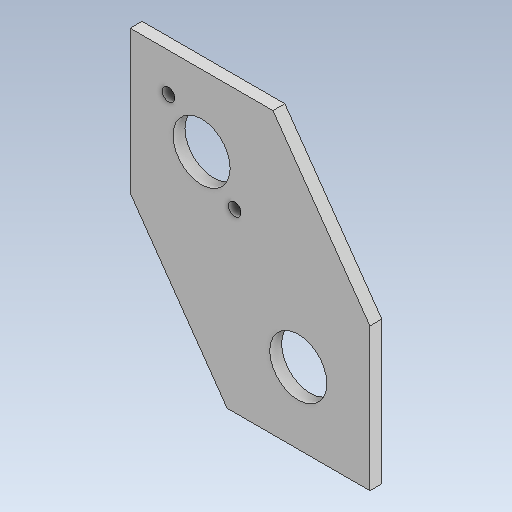
# Autodesk Inventor part: Motor and gearbox panel
Saved by Autodesk Inventor 2020.2 (Build 242310000, 310)
## iProperties
Created: 2020-02-27
Part Number: Motor and gearbox panel
Material: Generic
Document SubType Name: Modeling
Designer: deli
Density: 1 g/cm^3
Appearance: Default
Author: deli
Autodesk Inventor part; units mm, degrees
ref_plane "YZ Plane" through (0, 0, 0) normal (1, 0, 0) x (0, 1, 0)
ref_plane "XZ Plane" through (0, 0, 0) normal (0, 1, 0) x (-1, 0, 0)
ref_plane "XY Plane" through (0, 0, 0) normal (0, 0, 1) x (1, 0, 0)
sketch "Sketch1" plane through (0, 0, 0) normal (0, 0, 1) x (1, 0, 0)
  circle A0 centre (30.5438, 1.69) radius 1.7
  circle A1 centre (48.2215, -15.9877) radius 1.7
  line L0 (20.3327, -25.9449) -> (20.3327, 11.6471) projected
  circle A2 centre (39.3827, -7.1489) radius 7.62
  line L1 (39.3827, -7.1489) -> (121.2052, -7.1489) construction
  line L2 (20.3327, 11.9011) -> (58.4327, 11.9011)
  line L3 (39.3827, -7.1489) -> (118.6167, -7.1489) construction
  circle A3 centre (65.1936, -44.0106) radius 7.62
  line L4 (20.3327, 11.9011) -> (90.1827, 11.9011)
  line L5 (90.1827, 11.9011) -> (90.1827, -64.2989)
  line L6 (90.1827, -64.2989) -> (20.3327, -64.2989)
  line L7 (20.3327, -64.2989) -> (20.3327, 11.9011)
  circle A4 centre (65.1936, -44.0106) radius 18.9992
  line L8 (39.3827, -7.1489) -> (98.3795, -91.4051)
  line L9 (39.3827, -7.1489) -> (142.2405, -7.1489) construction
  line L10 (77.3997, -64.2989) -> (39.3827, -64.2989)
  line L11 (20.5867, 11.9011) -> (58.1787, 11.9011) projected
  line L12 (84.3087, -63.0098) -> (46.1944, -63.0098)
  line L13 (84.3087, -24.9302) -> (84.3087, -63.0098)
  line L14 (20.3327, -26.1989) -> (46.1944, -63.0098)
  line L15 (58.4327, 11.9011) -> (84.3087, -24.9302)
  point P0 (0, 0)
  dimension "d3" = 15.24
  dimension "d14" = 10.2112
  dimension "d17" = 27.8888
  dimension "d36" = 38.1
  dimension "d42" = 15.24
  dimension "d43" = 44.9999
  dimension "d51" = 69.85
  dimension "d52" = 76.2
  dimension "d53" = 37.9984
  dimension "d54" = 55
  dimension "d55" = 0
  dimension "d56" = 19.05
  dimension "d57" = 19.05
  dimension "d58" = 0
  constraints: 28 end point, 7 horizontal, 5 centre point, 3 parallel, 2 point on line, 1 coincident, 1 equal length, 1 midpoint, 1 perpendicular
  measures "d3" diameter of A2
  measures "d14" distance from line of L0 A0.centre
  measures "d17" distance from line of L0 A1.centre
  measures "d36" distance of L2.start L2.end
  measures "d42" diameter of A3
  measures "d43" distance of A3.centre L1.start
  measures "d51" distance of L5.end L6.end
  measures "d52" distance of L4.end L5.end
  measures "d53" diameter of A4
  measures "d54" angle of L8 L9
  measures "d55" distance from line of L8 A3.centre
  measures "d56" distance from line of L2 L1.start
  measures "d57" distance from line of L0 L1.start
  measures "d58" distance between parallel lines of L2 L11
extrude "Extrusion6" add sketch "Sketch1" along normal blind 3.175 contours L0 L7 L2 L15 L13 L12 L8 A4 L14 | A4 L8 A3 | A4 L8 L12 | A4 L8 A3
equation "\"d57\" = d56"
body "Solid6"
